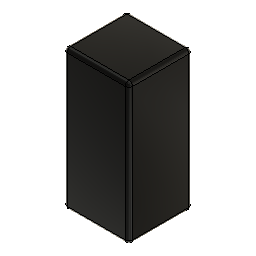
LiPo1300mAh4S45C v1 (Autodesk Fusion 360 design; units mm, degrees)
Autodesk Fusion 360 part; units mm, degrees
sketch "Sketch1" plane through (0, 0, 0) normal (0, 0, 1) x (1, 0, 0)
  line L0 (0, 0) -> (35, 0)
  line L1 (35, 0) -> (35, 34)
  line L2 (35, 34) -> (0, 34)
  line L3 (0, 34) -> (0, 0)
  dimension "d1" = 35
  dimension "d2" = 34
  constraint horizontal L0
  constraint vertical L1
  constraint horizontal L2
  constraint vertical L3
  constraint coincident L0.start L3.end
  measures "d1" distance of L0.start L0.end
  measures "d2" distance of L0.start L2.end
extrude "Extrude1" add sketch "Sketch1" along normal blind 75
fillet "Fillet1" radius 2 12 edges at (0, 17, 75) (17.5, 0, 75) (0, 0, 37.5) (35, 17, 75) (35, 34, 37.5) (17.5, 34, 0) (35, 0, 37.5) (17.5, 34, 75) (0, 17, 0) (35, 17, 0) (0, 34, 37.5) (17.5, 0, 0) 6 faces at (11.6667, 22.6667, 0) (0, 22.6667, 50) (23.3333, 34, 25) (11.6667, 0, 25) (11.6667, 22.6667, 75) (35, 11.3333, 50)
